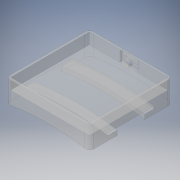
# Autodesk Inventor part: TrackDisplayBottom
Saved by Autodesk Inventor 2016 (Build 200138000, 138)
## iProperties
Created: 2016-05-05
Part Number: TrackDisplayBottom
Material: Generic
Document SubType Name: Modeling
Designer: xdlea
Density: 1 g/cm^3
Appearance: Default
Author: xdlea
Autodesk Inventor part; units mm, degrees
ref_plane "YZ Plane" through (0, 0, 0) normal (1, 0, 0) x (0, 1, 0)
ref_plane "XZ Plane" through (0, 0, 0) normal (0, 1, 0) x (-1, 0, 0)
ref_plane "XY Plane" through (0, 0, 0) normal (0, 0, 1) x (1, 0, 0)
sketch "Sketch1" plane through (0, 0, 0) normal (0, 1, 0) x (-1, 0, 0)
  circle A0 centre (0, 0) radius 25.4 construction
  line L0 (-28.575, 28.575) -> (28.575, 28.575)
  line L1 (28.575, 28.575) -> (28.575, -28.575)
  line L2 (28.575, -28.575) -> (-28.575, -28.575)
  line L3 (-28.575, -28.575) -> (-28.575, 28.575)
  line L4 (-28.575, 28.575) -> (28.575, -28.575) construction
  line L5 (28.575, 28.575) -> (-28.575, -28.575) construction
  line L6 (26.9875, 26.9875) -> (-26.9875, 26.9875)
  line L7 (-26.9875, 26.9875) -> (-26.9875, -26.9875)
  line L8 (-26.9875, -26.9875) -> (26.9875, -26.9875)
  line L9 (26.9875, -26.9875) -> (26.9875, 26.9875)
  line L10 (26.9875, 26.9875) -> (-26.9875, -26.9875) construction
  line L11 (-26.9875, 26.9875) -> (26.9875, -26.9875) construction
  dimension "d0" = 50.8
  dimension "d1" = 28.575
  dimension "d18" = 53.975
  constraints: 24 end point, 4 midpoint, 4 parallel, 3 perpendicular, 2 horizontal, 1 centre point, 1 coincident, 1 point on line
  measures "d0" diameter of A0
  measures "d1" distance from line of A0.centre L1
  measures "d18" distance of L7.end L8.end
extrude "Extrusion1" add sketch "Sketch1" along normal blind 7.62
extrude "Extrusion2" add sketch "Sketch1" against normal blind 3.175 contours L0 L1 L2 L3 | L9 L8 L7 L6
sketch "Sketch4" plane through (-25.4, -3.175, 28.575) normal (0, 0, 1) x (1, 0, 0)
  line L0 (53.975, 10.795) -> (53.975, 0) projected
  arc A0 (53.975, 0) -> (-3.175, 0) centre (25.4, -159.4644) ccw
  line L1 (-3.175, 0) -> (53.975, 0) construction
  arc A1 (53.975, -1.5875) -> (-3.175, -1.5875) centre (25.4, -161.0519) ccw
  arc A2 (53.975, -4.7625) -> (-3.175, -4.7625) centre (25.4, -164.2269) ccw
  line L2 (-3.175, -4.7625) -> (-3.175, -1.5875)
  line L3 (-3.175, -1.5875) -> (-3.175, 0)
  line L4 (53.975, -1.5875) -> (53.975, 0)
  line L5 (53.975, -4.7625) -> (53.975, -1.5875)
  point P0 (25.4, 2.54)
  dimension "d56" = 3.175
  dimension "d57" = 1.5875
  dimension "d58" = 2.54
  constraints: 10 end point, 7 point on circle, 3 centre point, 2 collinear, 2 equal radius, 2 horizontal alignment, 1 horizontal, 1 parallel, 1 point on line, 1 vertical
  measures "d56" distance of L5.start L4.start
  measures "d57" distance of L4.start L1.end
  measures "d58" distance from line of point (25.4, 2.54) L1
extrude "Extrusion11" add sketch "Sketch4" against normal up to surface (57.15 mm away)
extrude "Extrusion12" cut sketch "Sketch4" against normal blind 44.45 contours L4 A1 L3 A0
extrude "Extrusion13" cut sketch "Sketch4" against normal blind 38.1 contours L5 A2 L2 A1
extrude "Extrusion14" add sketch "Sketch4" against normal blind 12.7 contours L4 A1 L3 A0
extrude "Extrusion15" add sketch "Sketch4" against normal blind 19.05 contours L5 A2 L2 A1
fillet "Fillet6" radius 3.175 4 edges at (28.575, -0.1587, 28.575) (28.575, -0.1587, -28.575) (-28.575, -0.1587, 28.575) (-28.575, -0.1587, -28.575)
sketch "Sketch8" plane through (0, -167.4019, -28.575) normal (0, 0, -1) x (-1, 0, 0)
  line L0 (5, 168.4019) -> (-5, 168.4019)
  line L1 (-5, 168.4019) -> (-5, 167.4019)
  line L2 (-5, 167.4019) -> (6, 167.4019)
  line L3 (-26.9875, 167.4019) -> (26.9875, 167.4019) projected
  line L4 (6, 167.4019) -> (6, 174.4019)
  line L5 (6, 174.4019) -> (-5, 174.4019)
  line L6 (-5, 174.4019) -> (-5, 173.4019)
  line L7 (-5, 173.4019) -> (5, 173.4019)
  line L8 (5, 173.4019) -> (5, 168.4019)
  line L9 (-5, 173.4019) -> (-5, 168.4019)
  point P0 (0, 167.4019)
  point P1 (0, 168.4019)
  dimension "d68" = 1
  dimension "d74" = 1
  dimension "d75" = 1
  dimension "d76" = 7
  dimension "d77" = 10
  constraints: 18 end point, 3 perpendicular, 2 collinear, 2 horizontal, 2 vertical, 1 midpoint, 1 vertical alignment
  measures "d68" distance between parallel lines of L2 L0
  measures "d74" distance between parallel lines of L4 L8
  measures "d75" distance between parallel lines of L5 L7
  measures "d76" distance between parallel lines of L2 L5
  measures "d77" distance of L0.start L0.end
extrude "Extrusion16" cut sketch "Sketch8" against normal up to surface (1.5875 mm away) contours L8 L7 L6 L5 L4 L2 L1 L0
extrude "Extrusion17" add sketch "Sketch8" along normal blind 1 contours L0 L9 L7 L8
chamfer "Chamfer3" distance 1 angle 45 4 edges at (0, 6, -29.575) (-5, 3.5, -29.575) (0, 1, -29.575) (5, 3.5, -29.575)
sketch "Sketch9" plane through (-26.9875, 7.62, -26.9875) normal (0, 0, 1) x (1, 0, 0)
  circle A0 centre (26.9875, -4.12) radius 2.5
  line L0 (21.9875, -6.62) -> (21.9875, -1.62) projected
  point P0 (26.9875, -7.62)
  point P1 (21.9875, -4.12)
  dimension "d83" = 5
  constraints: 1 centre point, 1 horizontal alignment, 1 midpoint, 1 vertical alignment
  measures "d83" diameter of A0
extrude "Extrusion18" add sketch "Sketch9" along normal blind 2.6416
body "Solid1"
